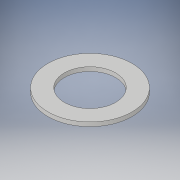
# Autodesk Inventor part: DireccionComplemento
Saved by Autodesk Inventor 2019 (Build 230136000, 136)
## iProperties
Created: 2020-04-23
Part Number: DireccionComplemento
Material: Generic
Document SubType Name: Modeling
Designer: Sergio
Density: 1 g/cm^3
Appearance: Default
Author: Sergio
Autodesk Inventor part; units mm, degrees
ref_plane "YZ Plane" through (0, 0, 0) normal (1, 0, 0) x (0, 1, 0)
ref_plane "XZ Plane" through (0, 0, 0) normal (0, 1, 0) x (-1, 0, 0)
ref_plane "XY Plane" through (0, 0, 0) normal (0, 0, 1) x (1, 0, 0)
sketch "Sketch1" plane through (0, 0, 0) normal (0, 1, 0) x (-1, 0, 0)
  circle A0 centre (0, 0) radius 12.5
  circle A1 centre (0, 0) radius 12.5
  circle A2 centre (0, 0) radius 20.5
  arc A3 (5.0111, -19.8781) -> (5.4667, 19.7577) centre (0, 0) ccw
  dimension "d0" = 41
  dimension "d1" = 25
  constraints: 4 centre point, 4 concentric, 2 coincident, 2 point on circle
  measures "d0" diameter of A2
  measures "d1" diameter of A0
extrude "Extrusion1" add sketch "Sketch1" along normal blind 2
body "Solid1"
